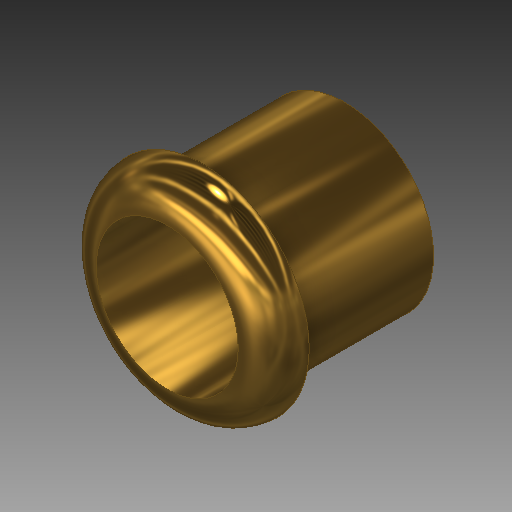
# Autodesk Inventor part: hole_big
Saved by Autodesk Inventor 2019 (Build 230136000, 136)
## iProperties
Created: 2019-11-15
Part Number: hole_big
Material: Латунь
Document SubType Name: Modeling
Designer: stepa
Density: 8.49 g/cm^3
Appearance: Латунь — полированная
Mass: 2.73299 g
Surface Area: 6.69576 cm^2
Volume: 0.321907 cm^3
Author: stepa
Autodesk Inventor part; units mm, degrees
ref_plane "YZ Plane" through (0, 0, 0) normal (1, 0, 0) x (0, 1, 0)
ref_plane "XZ Plane" through (0, 0, 0) normal (0, 1, 0) x (-1, 0, 0)
ref_plane "XY Plane" through (0, 0, 0) normal (0, 0, 1) x (1, 0, 0)
sketch "Эскиз1" plane through (0, 0, 0) normal (0, 0, 1) x (1, 0, 0)
  circle A0 centre (0, 0) radius 4
  circle A1 centre (0, 0) radius 5
  dimension "d0" = 8
  dimension "d1" = 10
  constraints: 2 centre point, 2 coincident
  measures "d0" diameter of A0
  measures "d1" diameter of A1
extrude "Выдавливание1" add sketch "Эскиз1" along normal blind 10
sketch "Эскиз2" plane through (0, 0, 10) normal (0, 0, 1) x (1, 0, 0)
  circle A0 centre (0, 0) radius 6
  circle A1 centre (0, 0) radius 5 projected
  dimension "d4" = 12
  constraints: 1 centre point, 1 coincident
  measures "d4" diameter of A0
extrude "Выдавливание2" add sketch "Эскиз2" against normal blind 2
fillet "Сопряжение1" radius 2 1 edges at (-6, 0, 10)
